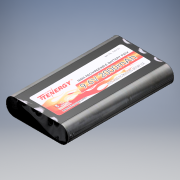
# Autodesk Inventor part: Tenergy NiMH Battery Pack 9.6V 2000mAh High Capacity Rechargeable RC Battery
Saved by Autodesk Inventor 2018 (Build 220112000, 112)
## iProperties
Created: 2018-11-09
Part Number: Tenergy NiMH Battery Pack 9.6V 2000mAh High Capacity Rechargeable RC Battery
Material: Generic
Document SubType Name: Modeling
Designer: Labs
Density: 1 g/cm^3
Appearance: Default
Author: Labs
Autodesk Inventor part; units mm, degrees
ref_plane "YZ Plane" through (0, 0, 0) normal (1, 0, 0) x (0, 1, 0)
ref_plane "XZ Plane" through (0, 0, 0) normal (0, 1, 0) x (-1, 0, 0)
ref_plane "XY Plane" through (0, 0, 0) normal (0, 0, 1) x (1, 0, 0)
sketch "Sketch1" plane through (0, 0, 0) normal (0, 0, 1) x (1, 0, 0)
  line L0 (-15.6633, 0) -> (44.0267, 0)
  line L1 (44.0267, 0) -> (44.0267, 16.51)
  line L2 (44.0267, 16.51) -> (-15.6633, 16.51)
  line L3 (-15.6633, 16.51) -> (-15.6633, 0)
  point P0 (0, 0)
  dimension "d0" = 16.51
  dimension "d1" = 59.69
  constraints: 8 end point, 2 parallel, 1 horizontal, 1 perpendicular
  measures "d0" distance of L0.end L1.end
  measures "d1" distance of L1.end L2.end
extrude "Extrusion1" add sketch "Sketch1" along normal mid plane 101.6
sketch "Sketch2" plane through (-9.3133, 16.51, 50.8) normal (0, 1, 0) x (1, 0, 0)
  line L0 (-6.35, 101.6) -> (-6.35, 0) projected
  line L1 (53.34, 0) -> (-6.35, 0) projected
  line L2 (53.34, 101.6) -> (53.34, 0) projected
  line L3 (-6.35, 101.6) -> (53.34, 101.6) projected
  line L4 (-6.35, 0) -> (-6.35, 101.6343) construction
  line L5 (-6.35, 101.6343) -> (53.34, 101.6343) construction
  line L6 (53.34, 101.6343) -> (53.34, 0) construction
  line L7 (53.34, 0) -> (-6.35, 0) construction
  constraints: 2 coincident, 2 other
sketch "Sketch3" plane through (-15.6633, 0, 50.8) normal (0, -1, 0) x (1, 0, 0)
  line L0 (59.69, -101.6) -> (59.69, 0) projected
  line L1 (0, 0) -> (59.69, 0) projected
  line L2 (0, 0) -> (0, -101.6) projected
  line L3 (59.69, -101.6) -> (0, -101.6) projected
  line L4 (0, 0) -> (59.69, 0) projected
  line L5 (59.69, 0) -> (59.6518, -101.6224) construction
  line L6 (59.6518, -101.6224) -> (0, -101.6) construction
  line L7 (0, -101.6) -> (0.0382, 0.0224) construction
  line L8 (0.0382, 0.0224) -> (59.69, 0) construction
  point P0 (15.6633, -50.8)
  constraints: 1 coincident, 2 other
sketch "Sketch4" plane through (44.0267, 0, 50.8) normal (0, 0, 1) x (1, 0, 0)
  line L0 (-59.69, 0) -> (0, 0) projected
  line L1 (0, 0) -> (0, 16.51) projected
  line L2 (0, 16.51) -> (-59.69, 16.51) projected
  line L3 (-59.69, 16.51) -> (-59.69, 0) projected
  line L4 (0, 16.51) -> (-59.69, 16.51) projected
  line L5 (-59.69, 16.51) -> (0.0244, 16.4214) construction
  line L6 (0.0244, 16.4214) -> (0, 0) construction
  line L7 (0, 0) -> (-59.7144, 0.0886) construction
  line L8 (-59.7144, 0.0886) -> (-59.69, 16.51) construction
  constraints: 1 coincident, 1 point on line, 2 other
sketch "Sketch5" plane through (0, 0, -50.8) normal (0, 0, -1) x (-1, 0, 0)
  line L0 (-44.0267, 0) -> (15.6633, 0) projected
  line L1 (15.6633, 0) -> (15.6633, 16.51) projected
  line L2 (15.6633, 16.51) -> (-44.0267, 16.51) projected
  line L3 (-44.0267, 16.51) -> (-44.0267, 0) projected
  line L4 (-44.0267, 16.51) -> (15.6633, 16.51) projected
  line L5 (-44.0267, 16.51) -> (15.6877, 16.4214) construction
  line L6 (15.6877, 16.4214) -> (15.6633, 0) construction
  line L7 (15.6633, 0) -> (-44.051, 0.0886) construction
  line L8 (-44.051, 0.0886) -> (-44.0267, 16.51) construction
  point P0 (0, 0)
  constraints: 1 coincident, 2 other
sketch "Sketch6" plane through (44.0267, 0, 50.8) normal (1, 0, 0) x (0, 0, -1)
  line L0 (101.6, 16.51) -> (0, 16.51) projected
  line L1 (0, 0) -> (0, 16.51) projected
  line L2 (101.6, 0) -> (0, 0) projected
  line L3 (101.6, 16.51) -> (101.6, 0) projected
  line L4 (101.6, 16.51) -> (0, 16.51) projected
  line L5 (0, 16.51) -> (101.6, 16.51) construction
  line L6 (101.6, 16.51) -> (101.6, 0) construction
  line L7 (101.6, 0) -> (0, 0) construction
  line L8 (0, 0) -> (0, 16.51) construction
  point P0 (50.8, 0)
  dimension "d174" = 101.6
  dimension "d175" = 16.51
  constraints: 1 coincident, 2 other
  measures "d174" distance of L0.start L0.end
  measures "d175" distance of L0.start L2.start
sketch "Sketch7" plane through (-15.6633, 0, 50.8) normal (-1, 0, 0) x (0, 0, 1)
  line L0 (-101.6, 16.51) -> (-101.6, 0) projected
  line L1 (-101.6, 16.51) -> (0, 16.51) construction
  line L2 (0, 16.51) -> (0, 0) construction
  line L3 (0, 0) -> (-101.6, 0) construction
  line L4 (-101.6, 0) -> (-101.6, 16.51) construction
  point P0 (-50.8, 0)
  constraints: 2 other
fillet "Fillet2" radius 7.62 4 edges at (44.0267, 16.51, 0) (44.0267, 0, 0) (-15.6633, 16.51, 0) (-15.6633, 0, 0)
decal "Decal1"
decal "Decal2"
decal "Decal3"
decal "Decal4"
decal "Decal5"
decal "Decal6"
body "Solid1"
